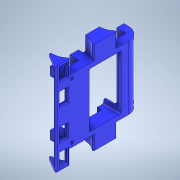
# Autodesk Inventor part: HullBottom
Saved by Autodesk Inventor 2021 (Build 250183000, 183)
## iProperties
Created: 2021-05-13
Part Number: HullBottom
Material: Generic
Document SubType Name: Modeling
Designer: ermoz
Density: 1 g/cm^3
Appearance: Default
Author: ermoz
Autodesk Inventor part; units mm, degrees
ref_plane "YZ Plane" through (0, 0, 0) normal (1, 0, 0) x (0, 1, 0)
ref_plane "XZ Plane" through (0, 0, 0) normal (0, 1, 0) x (-1, 0, 0)
ref_plane "XY Plane" through (0, 0, 0) normal (0, 0, 1) x (1, 0, 0)
sketch "Sketch1" plane through (0, 0, 0) normal (0, 1, 0) x (-1, 0, 0)
  circle A0 centre (0, 0) radius 15.5
  circle A1 centre (0, 50) radius 15.5
  circle A2 centre (0, 0) radius 17.5
  circle A3 centre (0, 50) radius 17.5
  line L0 (-13.5, 77.8812) -> (-13.5, 0)
  line L1 (5, 56) -> (-5, 56)
  line L2 (-5, 56) -> (-5, 44)
  line L3 (-5, 44) -> (5, 44)
  line L4 (5, 44) -> (5, 56)
  line L5 (5, 56) -> (-5, 44) construction
  line L6 (-5, 56) -> (5, 44) construction
  line L7 (5, -6) -> (-5, -6)
  line L8 (-5, -6) -> (-5, 6)
  line L9 (-5, 6) -> (5, 6)
  line L10 (5, 6) -> (5, -6)
  line L11 (5, -6) -> (-5, 6) construction
  line L12 (-5, -6) -> (5, 6) construction
  line L13 (5, 44) -> (5, 42)
  line L14 (5, 42) -> (0, 42)
  line L15 (0, 42) -> (0, 8)
  line L16 (0, 8) -> (5, 8)
  line L17 (5, 8) -> (5, 6)
  line L18 (5, 56) -> (5, 61)
  line L19 (5, 61) -> (-5, 61)
  line L20 (-15.5, -15.5) -> (32.2842, -15.5)
  line L21 (32.2842, -15.5) -> (32.2842, 82.5)
  line L22 (32.2842, 82.5) -> (-15.5, 82.5)
  line L23 (-15.5, 82.5) -> (-15.5, -15.5)
  line L24 (-15.5, 82.5) -> (10.4808, 67.5)
  line L25 (-15.5, 82.5) -> (14.5, 82.5) construction
  line L26 (10.4808, 67.5) -> (8.9808, 64.9019)
  line L27 (8.9808, 64.9019) -> (-17, 79.9019)
  line L28 (-17, 79.9019) -> (-15.5, 82.5)
  arc A4 (-13.5, 0) -> (0, -13.5) centre (0, 0) ccw
  line L29 (-10.5, 76.1491) -> (-10.5, 61)
  line L30 (-10.5, 61) -> (-5, 61)
  line L31 (0, -13.5) -> (5, -13.5)
  line L32 (5, -13.5) -> (5, -6)
  point P0 (-10.5, 64)
  point P1 (-13.5, 61.1355)
  point P2 (0, 17.5)
  point P3 (0, 32.5)
  point P4 (-13.5, 38.8645)
  point P5 (-13.5, 11.1355)
  dimension "d1" = 50
  dimension "d2" = 2
  dimension "d3" = 2
  dimension "d5" = 10
  dimension "d6" = 12
  dimension "d8" = 12
  dimension "d9" = 2
  dimension "d10" = 31
  dimension "d11" = 98
  dimension "d12" = 2
  dimension "d13" = 30
  dimension "d14" = 3
  dimension "d15" = 90
  dimension "d16" = 3
  dimension "d31" = 5
  dimension "d37" = 5
  constraints: 67 end point, 11 perpendicular, 6 horizontal, 6 parallel, 5 centre point, 4 midpoint, 4 tangent, 4 vertical, 3 equal length, 3 point on line, 2 coincident, 2 point on circle, 1 equal radius
  measures "d1" distance of A1.centre point (0, 0)
  measures "d2" radial gap between concentric circles of A0 A2
  measures "d3" radial gap between concentric circles of A1 A3
  measures "d5" distance of L3.end L2.end
  measures "d6" distance of L2.end L1.end
  measures "d8" distance of L7.end L8.end
  measures "d9" distance of L3.end L13.end
  measures "d10" diameter of A0
  measures "d11" distance of L22.end L20.start
  measures "d12" distance between parallel lines of L23 L0
  measures "d13" angle of L24 L25
  measures "d14" distance of L24.end L26.end
  measures "d15" angle of L24 L26
  measures "d16" distance between parallel lines of L0 L29
  measures "d31" distance of L1.start L18.end
  measures "d37" distance of L15.end L16.end
extrude "Extrusion1" add sketch "Sketch1" along normal mid plane 98 contours A2 L0 A3 L15 | L0 L27 L29 A3
extrude "Extrusion2" add sketch "Sketch1" along normal mid plane 68 contours L15 L16 L17 L9 L8 L7 L32 L31 A4 L0 A0 | A0 L0 A2 L15 | A3 L0 A1 L15 | A1 L0 L29 L30 L19 L18 L1 L2 L3 L13 L14 L15 | L0 A3 L29 A1
sketch "Sketch2" plane through (-5, -34, 61) normal (-1, 0, 0) x (0, 0, 1)
  line L0 (-5, 0) -> (-17, 0) projected
  line L1 (-17, 0) -> (-17, 68) projected
  line L2 (-5, 0) -> (-17, 0)
  line L3 (-17, 0) -> (-17, 9)
  line L4 (-17, 9) -> (-5, 9)
  line L5 (-5, 9) -> (-5, 0)
  line L6 (-5, 0) -> (-5, 68) projected
  line L7 (-5, 68) -> (-17, 68)
  line L8 (-17, 68) -> (-17, 59)
  line L9 (-17, 59) -> (-5, 59)
  line L10 (-5, 59) -> (-5, 68)
  line L11 (0, 0) -> (0, 68) projected
  line L12 (-67, 0) -> (-67, 68) projected
  line L13 (0, 9) -> (-67, 9)
  line L14 (-67, 9) -> (-67, 59)
  line L15 (-67, 59) -> (0, 59)
  line L16 (0, 59) -> (0, 9)
  point P0 (-61, 34)
  point P1 (0, 59)
  dimension "d21" = 9
  dimension "d22" = 9
  constraints: 24 end point, 6 parallel, 4 point on line, 3 horizontal, 3 perpendicular, 2 collinear
  measures "d21" distance of L2.end L3.end
  measures "d22" distance of L8.end L7.end
extrude "Extrusion3" cut sketch "Sketch2" against normal up to surface (15.5 mm away) contours L4 L1 L9 L6 | L6 L15 L11 L13 | L13 L12 L15 L1
sketch "Sketch3" plane through (10.5, -49, 76.1491) normal (-1, 0, 0) x (0, 0, 1)
  line L0 (0, 98) -> (0, 0) projected
  line L1 (0, 49) -> (-29.5622, 49)
  line L2 (-11.1491, 3) -> (-3.1491, 3)
  line L3 (-3.1491, 3) -> (-3.1491, 16)
  line L4 (-3.1491, 16) -> (-11.1491, 16)
  line L5 (-11.1491, 16) -> (-11.1491, 3)
  line L6 (-11.1491, 26) -> (-3.1491, 26)
  line L7 (-3.1491, 26) -> (-3.1491, 39)
  line L8 (-3.1491, 39) -> (-11.1491, 39)
  line L9 (-11.1491, 39) -> (-11.1491, 26)
  line L10 (-11.1491, 95) -> (-3.1491, 95)
  line L11 (-3.1491, 95) -> (-3.1491, 82)
  line L12 (-3.1491, 82) -> (-11.1491, 82)
  line L13 (-11.1491, 82) -> (-11.1491, 95)
  line L14 (-11.1491, 72) -> (-3.1491, 72)
  line L15 (-3.1491, 72) -> (-3.1491, 59)
  line L16 (-3.1491, 59) -> (-11.1491, 59)
  line L17 (-11.1491, 59) -> (-11.1491, 72)
  line L18 (-15.1491, 15) -> (-15.1491, 24) projected
  point P0 (-76.1491, 49)
  dimension "d46" = 13
  dimension "d47" = 8
  dimension "d48" = 10
  dimension "d49" = 33
  dimension "d57" = 4
  constraints: 34 end point, 8 symmetric about line, 4 parallel, 4 point on line, 3 horizontal, 2 perpendicular, 1 collinear, 1 midpoint
  measures "d46" distance of L2.end L3.end
  measures "d47" distance of L2.start L2.end
  measures "d48" distance from line of L1 L7.end
  measures "d49" distance from line of L3.end L1
  measures "d57" distance between parallel lines of L18 L5
extrude "Extrusion4" cut sketch "Sketch3" against normal through all
sketch "Sketch4" plane through (0, 49, 17.5) normal (-1, 0, 0) x (0, 0, 1)
  line L0 (24.5, -15) -> (24.5, -24) projected
  line L1 (-9.5, -83) -> (-9.5, -74) projected
  line L2 (24.5, -20) -> (-9.5, -20)
  line L3 (-9.5, -20) -> (-9.5, -78)
  line L4 (-9.5, -78) -> (24.5, -78)
  line L5 (24.5, -78) -> (24.5, -20)
  line L6 (24.5, -83) -> (15, -83) projected
  line L7 (24.5, -83) -> (-9.5, -83)
  line L8 (-9.5, -83) -> (-9.5, -78)
  line L9 (-9.5, -78) -> (24.5, -78)
  line L10 (24.5, -78) -> (24.5, -83)
  line L11 (-6.3645, -15) -> (-17.5, -15) projected
  line L12 (-9.5, -15) -> (24.5, -15)
  line L13 (24.5, -15) -> (24.5, -20)
  line L14 (24.5, -20) -> (-9.5, -20)
  line L15 (-9.5, -20) -> (-9.5, -15)
  line L16 (-23.5, -74) -> (-23.5, -24) projected
  line L17 (-23.5, -49) -> (15.7227, -49)
  point P0 (-17.5, -49)
  dimension "d32" = 5
  constraints: 26 end point, 6 parallel, 4 horizontal, 4 point on line, 3 perpendicular, 1 midpoint, 1 other
  measures "d32" distance of L9.end L6.start
extrude "Extrusion5" add sketch "Sketch4" along normal up to surface (5 mm away) contours L0 L2 L15 L11 L12 | L10 L6 L7 L1 L4
extrude "Extrusion6" cut sketch "Sketch4" against normal up to surface (10.5 mm away) contours L0 L5 L4 L1 L3 L2
sketch "Sketch5" plane through (0, 49, 0) normal (0, 1, 0) x (1, 0, 0)
  arc A0 (10.5, -64) -> (13.5, -61.1355) centre (0, -50) ccw projected
  circle A1 centre (0, -50) radius 17.5
  line L0 (10.5, -76.1491) -> (13.5, -77.8812) projected
  line L1 (10.5, -76.1491) -> (-7.0467, -66.0185)
  line L2 (10.5, -64) -> (10.5, -76.1491)
  line L3 (11.5, -72.489) -> (11.5, -65.964) projected
  point P0 (0, 0)
  constraints: 2 end point, 2 point on circle, 1 centre point, 1 coincident, 1 collinear, 1 vertical, 3 other
extrude "Extrusion7" add sketch "Sketch5" against normal blind 98 contours L2 L1 A1
extrude "Extrusion8" cut sketch "Sketch5" against normal blind 95 contours L2 L1 A1
extrude "Extrusion9" add sketch "Sketch5" against normal blind 3 contours L2 L1 A1
sketch "Sketch6" plane through (10.5, -25, -6) normal (-1, 0, 0) x (0, 0, 1)
  line L0 (48, -4) -> (14, -4) projected
  line L1 (14, 54) -> (48, 54) projected
  line L2 (14, -4) -> (48, -4)
  line L3 (48, -4) -> (48, 54)
  line L4 (48, 54) -> (14, 54)
  line L5 (14, 54) -> (14, -4)
  point P0 (6, 25)
  point P1 (14, 54)
  constraints: 8 end point, 2 parallel, 1 horizontal, 1 perpendicular
extrude "Extrusion10" cut sketch "Sketch6" against normal blind 3
fillet "Fillet1" radius 2 12 edges at (12, -29, 8) (2.75, -29, 8) (12, 29, 8) (2.75, 29, 8) (12, 29, 42) (2.75, 29, 42) (12, -29, 42) (2.75, -29, 42) (10.5, 25, 51.5) (10.5, 25, 1) (10.5, -25, 1) (10.5, -25, 51.5)
fillet "Fillet2" radius 1 8 edges at (13.5, 41.5, 38.8645) (13.5, 41.5, 61.1355) (13.5, 41.5, 11.1355) (13.5, -41.5, 11.1355) (13.5, -41.5, 38.8645) (13.5, -41.5, 61.1355) (-7.0467, 47.5, 66.0185) (-7.0467, -47.5, 66.0185)
fillet "Fillet3" radius 1 1 edges at (13.5, 0, 77.8812)
chamfer "Chamfer1" distance 1 angle 45 16 edges at (13.5, -46, 69) (13.5, -39.5, 73) (13.5, -33, 69) (13.5, -39.5, 65) (13.5, -23, 69) (13.5, -16.5, 65) (13.5, -10, 69) (13.5, -16.5, 73) (13.5, 16.5, 65) (13.5, 10, 69) (13.5, 23, 69) (13.5, 16.5, 73) (13.5, 39.5, 65) (13.5, 46, 69) (13.5, 39.5, 73) (13.5, 33, 69)
sketch "Sketch7" plane through (10.5, -46, 76.1491) normal (-1, 0, 0) x (0, 0, 1)
  line L0 (-15.1491, 12) -> (-20.1491, 12) projected
  line L1 (-15.1491, 12) -> (-11.1491, 12)
  line L2 (-11.1491, 12) -> (-11.1491, 21)
  line L3 (-11.1491, 21) -> (-15.1491, 21)
  line L4 (-15.1491, 21) -> (-15.1491, 12)
  line L5 (-11.1491, 0) -> (-11.1491, 13) projected
  line L6 (-15.1491, 21) -> (-20.1491, 21) projected
  line L7 (-15.1491, 80) -> (-11.1491, 80)
  line L8 (-11.1491, 80) -> (-11.1491, 71)
  line L9 (-11.1491, 71) -> (-15.1491, 71)
  line L10 (-15.1491, 71) -> (-15.1491, 80)
  line L11 (-15.1491, 80) -> (-12.1491, 80) projected
  line L12 (-15.1491, 71) -> (-15.1491, 80) projected
  line L13 (-20.1491, 71) -> (-15.1491, 71) projected
  line L14 (-11.1491, 79) -> (-11.1491, 92) projected
  point P0 (-76.1491, 46)
  constraints: 16 end point, 6 collinear, 4 parallel, 2 horizontal, 2 perpendicular
extrude "Extrusion11" add sketch "Sketch7" along normal up to surface (15.5 mm away)
fillet "Fillet4" radius 2 2 edges at (10.5, -25, 63) (10.5, 25, 63)
sketch "Sketch8" plane through (-5, 34, 6) normal (-1, 0, 0) x (0, 0, 1)
  line L0 (38, -68) -> (29, -68)
  line L1 (29, -68) -> (29, -59)
  line L2 (29, -59) -> (38, -59)
  line L3 (38, -59) -> (38, -68)
  line L4 (50, -68) -> (50, -59) projected
  line L5 (59, -59) -> (50, -59) projected
  line L6 (0, 0) -> (9, 0)
  line L7 (9, 0) -> (9, -9)
  line L8 (9, -9) -> (0, -9)
  line L9 (0, -9) -> (0, 0)
  line L10 (38, -9) -> (38, 0) projected
  line L11 (59, -9) -> (50, -9) projected
  line L12 (29, -68) -> (9, -68)
  line L13 (9, -68) -> (9, 0)
  line L14 (9, 0) -> (29, 0)
  line L15 (29, 0) -> (29, -68)
  point P0 (-6, -34)
  point P1 (9, -9)
  constraints: 24 end point, 6 parallel, 4 equal length, 3 horizontal, 3 perpendicular
extrude "Extrusion12" cut sketch "Sketch8" against normal up to surface (5 mm away) contours L12 L13 L7 L14 L15 L1
sketch "Sketch9" plane through (-5, -34, 56) normal (-1, 0, 0) x (0, 0, 1)
  circle A0 centre (4.5, 4.5) radius 1.5
  line L0 (9, 0) -> (0, 0) projected
  line L1 (0, 0) -> (0, 9) projected
  circle A1 centre (4.5, 63.5) radius 1.5
  line L2 (0, 59) -> (0, 68) projected
  line L3 (0, 68) -> (9, 68) projected
  point P0 (-56, 34)
  point P1 (4.5, 0)
  point P2 (0, 4.5)
  point P3 (0, 63.5)
  point P4 (4.5, 68)
  dimension "d63" = 3
  constraints: 4 midpoint, 2 centre point, 2 horizontal alignment, 2 vertical alignment, 1 equal radius
  measures "d63" diameter of A0
extrude "Extrusion13" cut sketch "Sketch9" against normal through all
sketch "Sketch10" plane through (-5, -34, -6) normal (-1, 0, 0) x (0, 0, 1)
  circle A0 centre (-4.5, 63.5) radius 1.5
  line L0 (0, 59) -> (0, 68) projected
  circle A1 centre (-4.5, 4.5) radius 1.5
  line L1 (0, 0) -> (0, 9) projected
  point P0 (6, 34)
  point P1 (0, 63.5)
  point P2 (0, 4.5)
  dimension "d66" = 3
  dimension "d67" = 4.5
  dimension "d68" = 3
  dimension "d69" = 4.5
  constraints: 2 centre point, 2 horizontal alignment, 2 midpoint
  measures "d66" diameter of A0
  measures "d67" distance from line of L0 A0.centre
  measures "d68" diameter of A1
  measures "d69" distance from line of L1 A1.centre
extrude "Extrusion14" cut sketch "Sketch10" against normal through all
body "Solid1"
